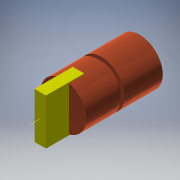
# Autodesk Inventor part: laser
Saved by Autodesk Inventor 2016 (Build 200138000, 138)
## iProperties
Created: 2016-05-31
Part Number: laser
Material: Generico
Document SubType Name: Modeling
Designer: Alfy Work
Density: 1 g/cm^3
Appearance: Default
Author: Alfy Work
Autodesk Inventor part; units mm, degrees
ref_plane "YZ Plane" through (0, 0, 0) normal (1, 0, 0) x (0, 1, 0)
ref_plane "XZ Plane" through (0, 0, 0) normal (0, 1, 0) x (-1, 0, 0)
ref_plane "XY Plane" through (0, 0, 0) normal (0, 0, 1) x (1, 0, 0)
sketch "Schizzo1" plane through (0, 0, 0) normal (0, 1, 0) x (-1, 0, 0)
  circle A0 centre (0, 0) radius 3
  dimension "d0" = 6
  constraints: 1 centre point, 1 coincident
  measures "d0" diameter of A0
extrude "Estrusione1" add sketch "Schizzo1" along normal blind 10
sketch "Schizzo2" plane through (0, 10, 0) normal (0, 1, 0) x (1, 0, 0)
  circle A0 centre (0, 0) radius 3 projected
  circle A1 centre (0, 0) radius 1.5
  dimension "d3" = 3
  constraints: 1 centre point, 1 coincident
  measures "d3" diameter of A1
extrude "Estrusione2" cut sketch "Schizzo2" against normal blind 1 contours A1
ref_plane "Piano di lavoro1" through (0, 5, 0) normal (0, -1, 0) x (1, 0, 0)
sketch "Schizzo3" plane through (0, 5, 0) normal (0, -1, 0) x (1, 0, 0)
  circle A0 centre (0, 0) radius 3 projected
  circle A1 centre (0, 0) radius 2.5
  dimension "d7" = 0.5
  constraints: 1 centre point
  measures "d7" radial gap between concentric circles of A0 A1
extrude "Estrusione3" cut sketch "Schizzo3" along normal blind 0.5
sketch "Schizzo4" plane through (0, 0, 0) normal (0, -1, 0) x (1, 0, 0)
  circle A0 centre (0, 0) radius 3 projected
  line L0 (-0.75, -3) -> (0.75, -3)
  line L1 (0.75, -3) -> (0.75, 3)
  line L2 (0.75, 3) -> (-0.75, 3)
  line L3 (-0.75, 3) -> (-0.75, -3)
  line L4 (-0.75, -3) -> (0.75, 3) construction
  line L5 (0.75, -3) -> (-0.75, 3) construction
  dimension "d10" = 1.5
  dimension "d11" = 6
  constraints: 12 end point, 2 midpoint, 2 parallel, 1 horizontal, 1 perpendicular
  measures "d10" distance of L2.end L1.end
  measures "d11" distance of L1.end L0.end
extrude "Estrusione4" add sketch "Schizzo4" along normal blind 3 and the other way blind 2 contours L1 A0 L3 | A0 L2 L1 | L1 L0 A0 | A0 L3 L2 | L0 L3 A0
